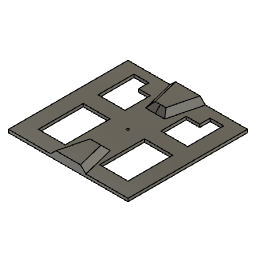
printable+top+piece (Autodesk Fusion 360 design; units mm, degrees)
Autodesk Fusion 360 part; units mm, degrees
sketch "Sketch1" plane through (0, 0, 0) normal (0, 0, 1) x (1, 0, 0)
  line L0 (0, 0) -> (101.6, 0)
  line L1 (101.6, 0) -> (101.6, 101.6)
  line L2 (101.6, 101.6) -> (0, 101.6)
  line L3 (0, 0) -> (0, 101.6)
  dimension "d1" = 101.6
  dimension "d2" = 101.6
  constraint coincident L0.start L3.start
  constraint horizontal L0
  constraint perpendicular L0 L1
  constraint perpendicular L1 L2
  constraint perpendicular L2 L3
  measures "d1" distance of L0.start L0.end
  measures "d2" distance of L0.end L1.end
extrude "Extrude1" add sketch "Sketch1" along normal blind 2.5
sketch "Sketch3" plane through (0, 0, 2.5) normal (0, 0, 1) x (-1, 0, 0)
  line L0 (-101.6, 0) -> (-101.6, -101.6)
  line L1 (-101.6, -101.6) -> (0, -101.6)
  line L2 (0, -101.6) -> (0, 0)
  line L3 (0, 0) -> (-101.6, 0)
  circle A0 centre (-50.8, -50.8) radius 1
  dimension "d11" = 2
  measures "d11" diameter of A0
extrude "Extrude3" add sketch "Sketch3" along normal blind 1.905 contours A0
sketch "Sketch4" plane through (0, 0, 2.5) normal (0, 0, 1) x (-1, 0, 0)
  line L0 (0, 0) -> (-5.08, 0)
  line L1 (-50.8, 0) -> (-38.1, 0)
  line L2 (-50.8, 0) -> (-63.5, 0)
  line L3 (-63.5, 0) -> (-57.15, -25.4)
  line L4 (-38.1, 0) -> (-44.45, -25.4)
  line L5 (-50.8, -25.4) -> (-44.45, -25.4)
  line L6 (-50.8, -25.4) -> (-57.15, -25.4)
  dimension "d35" = 25.4
  constraint coincident L0.start origin
  constraint horizontal L0
  measures "d35" distance of L1.start L5.start
sketch "Sketch6" plane through (0, 0, 2.5) normal (0, 0, 1) x (-1, 0, 0)
  line L0 (-50.8, -101.6) -> (-57.15, -101.6)
  line L1 (-50.8, -101.6) -> (-44.45, -101.6)
  line L2 (-44.45, -101.6) -> (-38.1, -101.6)
  line L3 (-57.15, -101.6) -> (-63.5, -101.6)
  line L4 (-38.1, -101.6) -> (-44.45, -76.2)
  line L5 (-57.15, -76.2) -> (-63.5, -101.6)
  line L6 (-50.8, -76.2) -> (-44.45, -76.2)
  line L7 (-50.8, -76.2) -> (-57.15, -76.2)
  dimension "d26" = 6.35
  dimension "d27" = 6.35
  dimension "d38" = 6.35
  dimension "d39" = 6.35
  dimension "d40" = 25.4
  constraint horizontal L0
  constraint parallel L0 L1
  constraint parallel L1 L2
  constraint parallel L0 L3
  measures "d26" distance of L0.start L0.end
  measures "d27" distance of L0.start L1.end
  measures "d38" distance of L1.end L2.end
  measures "d39" distance of L0.end L3.end
  measures "d40" distance of L0.start L6.start
extrude "Extrude6" add sketch "Sketch6" along normal blind 4.445
sketch "Sketch7" plane through (0, 0, 4.405) normal (0, 0, 1) x (-1, 0, 0)
  circle A0 centre (-50.8, -50.8) radius 1
  circle A1 centre (-50.8, -50.8) radius 1
  constraint concentric A0 A1
extrude "Extrude8" cut sketch "Sketch7" against normal blind 6.35
extrude "Extrude9" add sketch "Sketch4" along normal blind 4.445
chamfer "Chamfer3" distance 2.2225 angle 45 8 edges at (60.325, 12.7, 6.945) (60.325, 12.7, 2.5) (41.275, 12.7, 2.5) (41.275, 12.7, 6.945) (47.625, 25.4, 6.945) (53.975, 25.4, 6.945) (47.625, 25.4, 2.5) (53.975, 25.4, 2.5) measured on face at (50.8, 8.4667, 6.945) measured on face at (16.6, 50.8, 2.5) measured on face at (16.6, 50.8, 2.5) measured on face at (50.8, 8.4667, 6.945) measured on face at (50.8, 8.4667, 6.945) measured on face at (50.8, 8.4667, 6.945) measured on face at (16.6, 50.8, 2.5) measured on face at (16.6, 50.8, 2.5)
chamfer "Chamfer4" distance 2.2225 angle 45 8 edges at (53.975, 76.2, 6.945) (47.625, 76.2, 6.945) (53.975, 76.2, 2.5) (47.625, 76.2, 2.5) (41.275, 88.9, 6.945) (60.325, 88.9, 6.945) (60.325, 88.9, 2.5) (41.275, 88.9, 2.5) measured on face at (50.8, 93.1333, 6.945) measured on face at (50.8, 93.1333, 6.945) measured on face at (14.2382, 43.0742, 2.5) measured on face at (14.2382, 43.0742, 2.5) measured on face at (50.8, 93.1333, 6.945) measured on face at (50.8, 93.1333, 6.945) measured on face at (14.2382, 43.0742, 2.5) measured on face at (14.2382, 43.0742, 2.5)
sketch "Sketch5" plane through (0, 0, 2.5) normal (0, 0, 1) x (-1, 0, 0)
  line L0 (-12.7, -50.8) -> (-12.7, -25.4)
  line L1 (-12.7, -25.4) -> (-12.7, -12.7)
  line L2 (-12.7, -12.7) -> (-25.4, -12.7)
  line L3 (-34.7636, -50.8) -> (-12.7, -50.8)
  line L4 (-76.2, -12.7) -> (-88.9, -12.7)
  line L5 (-88.9, -12.7) -> (-88.9, -50.8)
  line L6 (-88.9, -50.8) -> (-66.04, -50.8)
  line L7 (-12.7, -93.98) -> (-12.7, -76.2)
  line L8 (-12.7, -76.2) -> (-12.7, -63.5)
  line L9 (-12.7, -63.5) -> (-35.56, -63.5)
  line L10 (-35.56, -63.5) -> (-35.56, -78.74)
  line L11 (-25.4, -93.98) -> (-12.7, -93.98)
  line L12 (-88.9, -63.5) -> (-66.04, -63.5)
  line L13 (-66.04, -63.5) -> (-66.04, -78.74)
  line L14 (-77.47, -85.121) -> (-77.47, -93.98)
  line L15 (-77.47, -93.98) -> (-88.9, -93.98)
  line L16 (-88.9, -93.98) -> (-88.9, -63.5)
  line L17 (-66.04, -78.74) -> (-66.04, -81.28)
  line L18 (-35.56, -78.74) -> (-35.56, -81.28)
  line L19 (-25.4, -85.121) -> (-35.56, -85.121)
  line L20 (-35.56, -85.121) -> (-35.56, -81.28)
  line L21 (-66.04, -85.121) -> (-77.47, -85.121)
  line L22 (-66.04, -85.121) -> (-66.04, -81.28)
  line L23 (-25.4, -85.121) -> (-25.4, -93.98)
  line L24 (-25.4, -12.7) -> (-33.02, -12.7)
  line L25 (-68.58, -12.7) -> (-76.2, -12.7)
  line L26 (-34.7636, -50.8) -> (-35.56, -50.8)
  line L27 (-35.56, -50.8) -> (-35.56, -12.7)
  line L28 (-66.04, -50.8) -> (-64.77, -50.8)
  line L29 (-64.77, -50.8) -> (-64.77, -12.7)
  line L30 (-64.77, -12.7) -> (-68.58, -12.7)
  line L31 (-35.56, -12.7) -> (-33.02, -12.7)
  constraint vertical L0
  constraint parallel L0 L1
  constraint perpendicular L0 L2
  constraint perpendicular L0 L3
  constraint perpendicular L4 L5
  constraint vertical L7
  constraint parallel L7 L8
  constraint perpendicular L8 L9
  constraint perpendicular L9 L10
  constraint perpendicular L7 L11
  constraint horizontal L12
  constraint perpendicular L12 L13
  constraint perpendicular L12 L14
  constraint perpendicular L14 L15
  constraint perpendicular L12 L16
  constraint perpendicular L20 L21
  constraint perpendicular L6 L29
extrude "Extrude7" cut sketch "Sketch5" against normal blind 10.16
